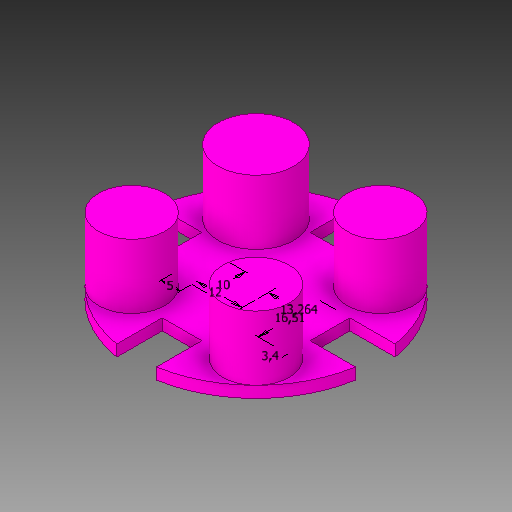
# Autodesk Inventor part: Circuit
Saved by Autodesk Inventor 2018 (Build 220112000, 112)
## iProperties
Created: 2018-01-14
Part Number: Circuit
Material: Generic
Document SubType Name: Modeling
Designer: Suchanek
Density: 1 g/cm^3
Appearance: Default
Author: Suchanek
Autodesk Inventor part; units mm, degrees
ref_plane "YZ Plane" through (0, 0, 0) normal (1, 0, 0) x (0, 1, 0)
ref_plane "XZ Plane" through (0, 0, 0) normal (0, 1, 0) x (-1, 0, 0)
ref_plane "XY Plane" through (0, 0, 0) normal (0, 0, 1) x (1, 0, 0)
sketch "Sketch4" plane through (0, 0, 0) normal (0, 1, 0) x (-1, 0, 0)
  circle A0 centre (0, 0) radius 32
  dimension "d48" = 64
  constraints: 1 centre point, 1 coincident
  measures "d48" diameter of A0
extrude "Extrusion1" add sketch "Sketch4" along normal blind 3
sketch "Sketch11" plane through (0, 0, 0) normal (0, -1, 0) x (1, 0, 0)
  point P0 (0, 0)
sketch "Sketch12" plane through (0, 3, 0) normal (0, 1, 0) x (1, 0, 0)
  circle A0 centre (16.4402, -16.4402) radius 8.75
  circle A1 centre (-15.5563, 15.5563) radius 10
  circle A2 centre (-16.4402, -16.4402) radius 8.75
  circle A3 centre (16.4402, 16.4402) radius 8.75
  line L0 (0, 0) -> (-4.7389, -4.7389)
  line L1 (0, 0) -> (6.7018, 0) construction
  line L2 (0, 0) -> (4.7389, -4.7389)
  dimension "d105" = 17.5
  dimension "d106" = 20
  dimension "d107" = 17.5
  dimension "d108" = 17.5
  dimension "d109" = 135
  dimension "d110" = 23.25
  dimension "d111" = 22
  dimension "d112" = 23.25
  constraints: 6 end point, 4 centre point, 4 point on line, 1 equal length, 1 horizontal, 1 perpendicular, 1 symmetric about line
  measures "d105" diameter of A0
  measures "d106" diameter of A1
  measures "d107" diameter of A2
  measures "d108" diameter of A3
  measures "d109" angle of L0 L1
  measures "d110" distance of L0.start A3.centre
  measures "d111" distance of L0.start A1.centre
  measures "d112" distance of L0.start A0.centre
extrude "Extrusion6" add sketch "Sketch12" along normal blind 17
sketch "Sketch13" plane through (0, 0, 0) normal (0, -1, 0) x (1, 0, 0)
  line L0 (5.25, -39.5664) -> (-5.25, -39.5664)
  line L1 (-5.25, -39.5664) -> (-5.25, -19.5664)
  line L2 (-5.25, -19.5664) -> (5.25, -19.5664)
  line L3 (5.25, -19.5664) -> (5.25, -39.5664)
  line L4 (0, 0) -> (0, -5.0055)
  arc A0 (5.25, -31.5664) -> (-5.25, -31.5664) centre (0, 0) ccw
  arc A1 (-5.25, -31.5664) -> (5.25, -31.5664) centre (0, 0) ccw
  circle A2 centre (0, 0) radius 32 projected
  line L5 (39.5664, 5.25) -> (39.5664, -5.25)
  line L6 (39.5664, -5.25) -> (19.5664, -5.25)
  line L7 (19.5664, -5.25) -> (19.5664, 5.25)
  line L8 (19.5664, 5.25) -> (39.5664, 5.25)
  arc A3 (31.5664, -5.25) -> (31.5664, 5.25) centre (0, 0) ccw
  line L9 (-5.25, 39.5664) -> (5.25, 39.5664)
  line L10 (5.25, 39.5664) -> (5.25, 19.5664)
  line L11 (5.25, 19.5664) -> (-5.25, 19.5664)
  line L12 (-5.25, 19.5664) -> (-5.25, 39.5664)
  arc A4 (5.25, 31.5664) -> (-5.25, 31.5664) centre (0, 0) ccw
  line L13 (-39.5664, -5.25) -> (-39.5664, 5.25)
  line L14 (-39.5664, 5.25) -> (-19.5664, 5.25)
  line L15 (-19.5664, 5.25) -> (-19.5664, -5.25)
  line L16 (-19.5664, -5.25) -> (-39.5664, -5.25)
  arc A5 (-31.5664, 5.25) -> (-31.5664, -5.25) centre (0, 0) ccw
  dimension "d115" = 10.5
  dimension "d116" = 20
  dimension "d117" = 12
  dimension "d118" = 0
  dimension "d121" = 360
  constraints: 34 end point, 10 point on circle, 8 point on line, 5 centre point, 3 coincident, 2 parallel, 1 horizontal, 1 perpendicular, 1 vertical, 48 other
  measures "d115" distance of L1.end L2.end
  measures "d116" distance between parallel lines of L2 L0
  measures "d117" distance of L2.end A0.start
  measures "d118" radial gap between concentric circles of A2 A0
extrude "Extrusion7" cut sketch "Sketch13" against normal blind 17 contours A1 L1 L2 L3 | L6 L7 L8 A0 | A0 L14 L15 L16 | A0 L10 L11 L12
sketch "Sketch14" plane through (0, 0, 0) normal (0, -1, 0) x (1, 0, 0)
  line L0 (13.264, -8.255) -> (16.664, -8.255)
  line L1 (16.664, -8.255) -> (16.664, 8.255)
  line L2 (16.664, 8.255) -> (13.264, 8.255)
  line L3 (13.264, 8.255) -> (13.264, -8.255)
  line L4 (0, 0) -> (2.53, 0)
  line L5 (-17, -5) -> (-12, -5)
  line L6 (-12, -5) -> (-12, 5)
  line L7 (-12, 5) -> (-17, 5)
  line L8 (-17, 5) -> (-17, -5)
  dimension "d125" = 13.264
  dimension "d126" = 16.51
  dimension "d127" = 3.4
  dimension "d128" = 12
  dimension "d129" = 5
  dimension "d130" = 10
  constraints: 18 end point, 4 parallel, 3 horizontal, 2 perpendicular, 2 other
  measures "d125" distance from line of L4.start L3
  measures "d126" distance of L2.end L0.start
  measures "d127" distance of L1.end L2.end
  measures "d128" distance from line of L4.start L6
  measures "d129" distance of L6.end L7.end
  measures "d130" distance of L5.end L6.end
body "Solid1"
